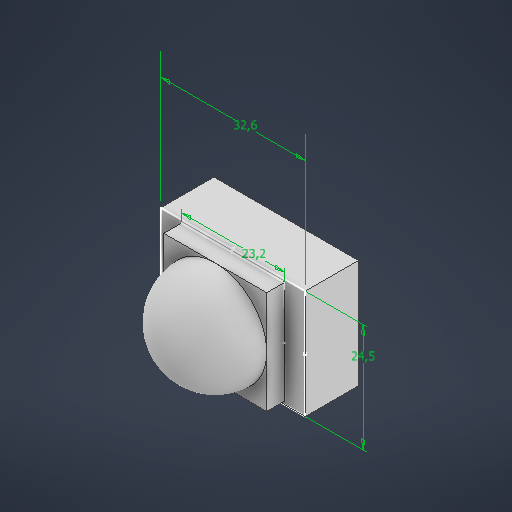
# Autodesk Inventor part: pir
Saved by Autodesk Inventor 2025.2 (Build 292293000, 293)
## iProperties
Created: 2024-12-17
Part Number: pir
Material: Generic
Document SubType Name: Modeling
Designer: antem
Density: 1 g/cm^3
Appearance: Default
Author: antem
Autodesk Inventor part; units mm, degrees
ref_plane "YZ Plane" through (0, 0, 0) normal (1, 0, 0) x (0, 1, 0)
ref_plane "XZ Plane" through (0, 0, 0) normal (0, 1, 0) x (-1, 0, 0)
ref_plane "XY Plane" through (0, 0, 0) normal (0, 0, 1) x (1, 0, 0)
sketch "Sketch1" plane through (0, 0, 0) normal (0, 1, 0) x (-1, 0, 0)
  line L0 (16.3, 12.25) -> (-16.3, 12.25)
  line L1 (-16.3, 12.25) -> (-16.3, -12.25)
  line L2 (-16.3, -12.25) -> (16.3, -12.25)
  line L3 (16.3, -12.25) -> (16.3, 12.25)
  line L4 (11.6, 11.6) -> (-11.6, 11.6)
  line L5 (-11.6, 11.6) -> (-11.6, -11.6)
  line L6 (-11.6, -11.6) -> (11.6, -11.6)
  line L7 (11.6, -11.6) -> (11.6, 11.6)
  point P0 (0, 0)
  point P1 (-11.6, 0)
  point P2 (-16.3, 0)
  point P3 (0, 12.25)
  point P4 (0, 11.6)
  dimension "d0" = 32.6
  dimension "d1" = 24.5
  dimension "d2" = 23.2
  constraints: 16 end point, 4 midpoint, 4 parallel, 3 perpendicular, 2 horizontal, 2 horizontal alignment, 2 vertical alignment
  measures "d0" distance of L0.start L0.end
  measures "d1" distance of L0.end L1.end
  measures "d2" distance of L4.start L4.end
extrude "Extrusion1" add sketch "Sketch1" along normal blind 12 contours L3 L2 L1 L0 | L7 L6 L5 L4
extrude "Extrusion2" add sketch "Sketch1" against normal blind 4 contours L7 L6 L5 L4
sketch "Sketch2" plane through (0, -4, 0) normal (0, -1, 0) x (1, 0, 0)
  line L0 (11.6, 11.6) -> (-11.6, 11.6) projected
  line L1 (0, 11.6) -> (0, -11.6)
  line L2 (11.6, -11.6) -> (-11.6, -11.6) projected
  arc A0 (0, -11.6) -> (0, 11.6) centre (0, 0) ccw
  constraints: 3 midpoint, 2 end point, 2 point on circle, 1 centre point, 1 coincident
revolve "Revolution1" add sketch "Sketch2" angle 360 about axis through (0, -4, 11.6) along (0, 0, -1)
body "Solid1"
